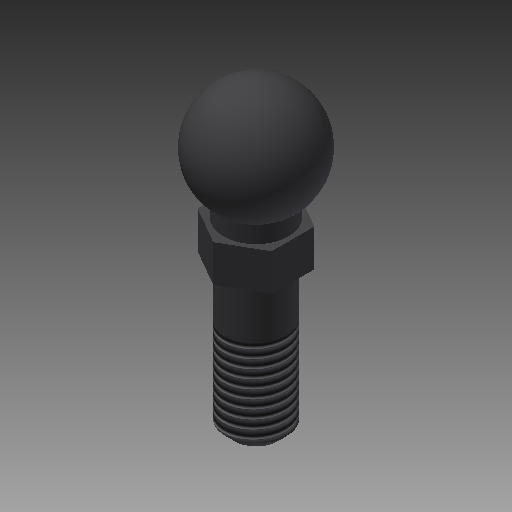
# Autodesk Inventor part: LHSA 14 Body2
Saved by Autodesk Inventor 2018 (Build 220112000, 112)
## iProperties
Category: PARTsolutions
Company: IKO
Created: 2017-09-07
Part Number: LHSA 14 Body2
Catalog Web Link: www.cadenas.de
Description: LHSA B2-
Vendor: IKO
Document SubType Name: Modeling
Designer: psAdmin
Manufacturer: IKO
Mass: 16.2172 g
Surface Area: 42.6268 cm^2
Volume: 16.2172 cm^3
Density: 1 g/cm^3
Material: 一般
Appearance: PSOLRGB-128-128-128
PSOL_IDENT_0: {$CADENAS_DATA\23d-libs\iko\iko_bearings\l_balls\lhsa_body2.prj},169 {VTYP=3D},{NB=LHSA 14 Body2},{L
PSOL_IDENT_1: INA=LHSA 14 Body2},{NN=LHSA B2},{DATE=13.10.2016 10:02:12},{GEOMDATE=05.12.2007 13:50:00},{VERSION=}
PSOL_IDENT_2: ,{LINEID=90},{LINESUBID=-1},{WBVAR=}  {NB=LHSA 14 Body2},{LINA=LHSA 14 Body2},{KT=DUMMY},{IDNR=},{OR
PSOL_IDENT_3: DER=LHSA 14},{RID=G_80},{STDRT=14},{DESCR=LHSA},{TRNUMBER=},{PAST=A},{REST=O},{MASS=260},{S=M14x2},{
PSOL_IDENT_4: KDM=11.546},{NDM=14.000},{P1=2.000},{V=14},{D=38},{L=76.0},{L1=57},{L2=30},{SL1=8.0},{W=22},{W1=22},
PSOL_IDENT_5: {W2=22},{D1=20.0},{D2=25},{LL=72.0},{P=17.0},{LL1=22.5},{LL2=33.5},{LL3=22.0},{SDK=25.400},{V1=15.0}
PSOL_IDENT_6: ,{D3=15.0000},{D4=28.2138},{D5=34.0},{D6=34.00},{L3=71.2350},{L4=35.1132},{L5=38.0},{L12=39.3932},{B=
PSOL_IDENT_7: 12.0},{B1=7.0},{B2=12.0},{B3=15.0},{B4=16.8},{B5=21.8000},{LL4=8.5},{LL5=12.7},{CB=0.0},{CC=1.0},{E=
PSOL_IDENT_8: 0},{F=0.0},{C1=1.5825},{C2=2.0},{R1=5},{R2=50.6010},{R3=20.0},{R4=1.5},{CS=14600},{SS1=11.546},{S1=1
PSOL_IDENT_9: 4},{LX=32},{LX1=36.6},{BL=3},{SC=1}
NN: LHSA B2
NB: LHSA 14 Body2
NBSYN: $ORDER. Body2
LINA: LHSA 14 Body2
ORDER: LHSA 14
RID: G_80
STDRT: 14
DESCR: LHSA
PAST: A
REST: O
MASS: 260
S: M14x2
NDM: 14.000
P1: 2.000
V: 14
D: 38
L: 76.0
L1: 57
L2: 30
SL1: 8.0
W: 22
W1: 22
W2: 22
D1: 20.0
D2: 25
LL: 72.0
P: 17.0
LL1: 22.5
LL2: 33.5
LL3: 22.0
SDK: 25.400
V1: 15.0
D3: 15.0000
D4: 28.2138
D5: 34.0
D6: 34.00
L3: 71.2350
L4: 35.1132
L5: 38.0
L12: 39.3932
B: 12.0
B1: 7.0
B2: 12.0
B3: 15.0
B4: 16.8
B5: 21.8000
LL4: 8.5
LL5: 12.7
CB: 0.0
CC: 1.0
E: 0
F: 0.0
C1: 1.5825
C2: 2.0
R1: 5
R2: 50.6010
R3: 20.0
R4: 1.5
CS: 14600
SS1: 11.546
S1: 14
LX: 32
LX1: 36.6
BL: 3
SC: 1
SUPPLIER: IKO
ARTICLENO: LHSA 14 Body2
BOMINFO: LHSA 14 Body2
CREATOR: CADENAS GmbH
Title: LHSA 14 Body2
Author: Cadenas PARTsolutions
Autodesk Inventor part; units mm, degrees
sketch "Sketch_2" plane through (0, 0, 0) normal (0, 0, 1) x (1, 0, 0)
  line L0 (0, -33.5) -> (0, 35.2)
  arc A0 (8.0777, 12.7) -> (0, 35.2) centre (0, 22.5) ccw
  line L1 (8.0777, 12.7) -> (7.5, 12.7)
  line L2 (7.5, 12.7) -> (7.5, 8.5)
  line L3 (7.5, 8.5) -> (11.05, 8.5)
  line L4 (11.05, 8.5) -> (11.05, 0)
  line L5 (11.05, 0) -> (7, 0)
  line L6 (7, 0) -> (7, -31.5)
  line L7 (7, -31.5) -> (5, -33.5)
  line L8 (5, -33.5) -> (0, -33.5)
  line L9 (0, -33.5) -> (0, 35.2)
  constraints: 20 end point, 2 point on circle, 1 centre point
revolve "Revolution1" add sketch "Sketch_2" angle 360 about axis through (0, -33.5, 0) along (0, -1, 0)
thread "Thread1" size "M14x2" class "6g" standard "ISO Metric profile" length 20
sketch "Sketch_3" plane through (0, 8.5, 0) normal (0, 1, 0) x (1, 0, 0)
  line L0 (-17, -17) -> (17, -17)
  line L1 (17, -17) -> (17, 17)
  line L2 (17, 17) -> (-17, 17)
  line L3 (-17, 17) -> (-17, -17)
  line L4 (-8.5, -4.9075) -> (0, -9.815)
  line L5 (0, -9.815) -> (8.5, -4.9075)
  line L6 (8.5, -4.9075) -> (8.5, 4.9075)
  line L7 (8.5, 4.9075) -> (0, 9.815)
  line L8 (0, 9.815) -> (-8.5, 4.9075)
  line L9 (-8.5, 4.9075) -> (-8.5, -4.9075)
  constraints: 20 end point
extrude "Extrusion1" cut sketch "Sketch_3" against normal blind 8.5
ref_plane "IP1_XY" through (0, 22.5, 0) normal (0, 0, -1) x (1, 0, 0)
ref_plane "IP1_YZ" through (0, 22.5, 0) normal (1, 0, 0) x (0, -1, 0)
ref_plane "IP1_ZX" through (0, 22.5, 0) normal (0, -1, 0) x (0, 0, -1)
body "Solid1"
